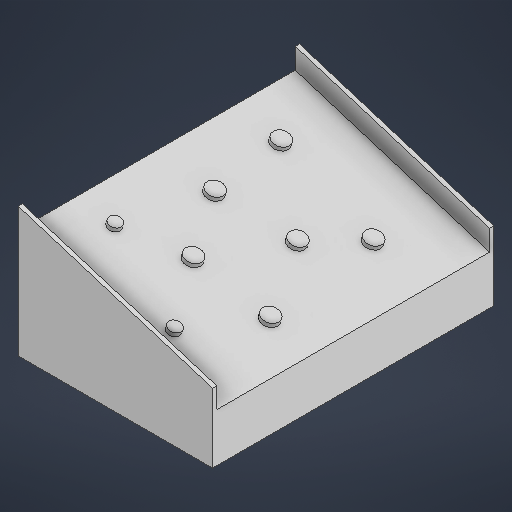
# Autodesk Inventor part: newcollection
Saved by Autodesk Inventor 2026.2 (Build 302298000, 298)
## iProperties
Created: 2026-04-15
Part Number: newcollection
Material: Generic
Document SubType Name: Modeling
Designer: danda
Density: 1 g/cm^3
Appearance: Default
Author: danda
Autodesk Inventor part; units mm, degrees
ref_plane "YZ Plane" through (0, 0, 0) normal (1, 0, 0) x (0, 1, 0)
ref_plane "XZ Plane" through (0, 0, 0) normal (0, 1, 0) x (-1, 0, 0)
ref_plane "XY Plane" through (0, 0, 0) normal (0, 0, 1) x (1, 0, 0)
sketch "Sketch1" plane through (0, 0, 0) normal (0, 0, 1) x (1, 0, 0)
  line L0 (-69.9828, 93.1946) -> (155.0172, 93.1946)
  line L1 (155.0172, 93.1946) -> (155.0172, 43.1946)
  line L2 (155.0172, 43.1946) -> (-69.9828, 43.1946)
  line L3 (-69.9828, 43.1946) -> (-69.9828, 93.1946)
  line L4 (-69.9828, 93.1946) -> (-69.9828, 163.1946)
  line L5 (-69.9828, 163.1946) -> (155.0172, 93.1946)
  line L6 (-74.9828, 93.1946) -> (-74.9828, 38.1946)
  line L7 (-74.9828, 38.1946) -> (160.0172, 38.1946)
  line L8 (160.0172, 38.1946) -> (160.0172, 96.8754)
  line L9 (-74.9828, 93.1946) -> (-74.9828, 169.9865)
  line L10 (-74.9828, 169.9865) -> (160.0172, 96.8754)
  line L11 (-69.9828, 163.1946) -> (-74.9828, 163.1946)
  line L12 (155.0172, 93.1946) -> (160.0172, 93.1946)
  line L13 (-69.9828, 93.1946) -> (-74.9828, 93.1946)
  point P0 (0, 0)
  dimension "d0" = 225
  dimension "d1" = 50
  dimension "d2" = 70
  dimension "d3" = 5
  dimension "d4" = 5
  constraints: 28 end point, 3 parallel, 3 perpendicular, 2 point on line, 1 collinear, 1 horizontal, 1 vertical, 1 other
  measures "d0" distance of L1.end L2.end
  measures "d1" distance of L0.end L1.end
  measures "d2" distance of L0.start L4.end
  measures "d3" distance between parallel lines of L3 L6
  measures "d4" distance between parallel lines of L4 L9
extrude "Extrusion1" add sketch "Sketch1" along normal blind 340 contours L13 L9 L11 L4 | L3 L2 L1 L12 L8 L7 L6 L13 | L5 L11 L9 L10 L8 L12
extrude "Extrusion2" add sketch "Sketch1" along normal blind 340 contours L4 L5 L0 | L0 L1 L2 L3
extrude "Extrusion3" cut sketch "Sketch1" along normal blind 335 contours L4 L5 L0 | L0 L1 L2 L3
extrude "Extrusion4" add sketch "Sketch1" along normal blind 5 contours L4 L5 L0 | L0 L1 L2 L3
sketch "Sketch2" plane through (-74.9828, 169.9865, 340) normal (0.2970666, 0.9548568, 0) x (0.9548568, -0.2970666, 0)
  line L0 (42.4399, 335) -> (42.4399, 5) projected
  circle A0 centre (42.4399, 75.4833) radius 7.5
  circle A1 centre (53.1004, 265.9353) radius 10
  circle A2 centre (108.208, 107.2253) radius 10
  circle A3 centre (63.1004, 176.4405) radius 10
  circle A4 centre (158.9071, 36.2466) radius 7.5
  circle A5 centre (180.5093, 255.9353) radius 10
  circle A6 centre (144.7995, 198.4836) radius 10
  circle A7 centre (195.4985, 117.2253) radius 10
  point P0 (122.0951, 340)
  dimension "d13" = 15
  dimension "d14" = 20
  dimension "d15" = 20
  dimension "d16" = 20
  dimension "d17" = 15
  dimension "d18" = 20
  dimension "d19" = 20
  dimension "d20" = 20
  constraints: 8 centre point, 1 point on line
  measures "d13" diameter of A0
  measures "d14" diameter of A1
  measures "d15" diameter of A2
  measures "d16" diameter of A3
  measures "d17" diameter of A4
  measures "d18" diameter of A5
  measures "d19" diameter of A6
  measures "d20" diameter of A7
extrude "Extrusion5" add sketch "Sketch2" along normal blind 5
sketch "Sketch3" plane through (0, 0, 340) normal (0, 0, 1) x (1, 0, 0)
  line L0 (-69.9828, 163.1946) -> (158.5319, 92.1011)
  line L1 (160.0172, 96.8754) -> (-74.9828, 169.9865) projected
  line L2 (-75.9241, 144.0974) -> (155.0172, 72.249)
  line L3 (-69.9828, 163.1946) -> (-69.9828, 142.249)
  line L4 (-69.9828, 43.1946) -> (-69.9828, 163.1946) projected
  line L5 (155.0172, 43.1946) -> (155.0172, 93.1946) projected
  line L6 (155.0172, 93.1946) -> (155.0172, 72.249)
  line L7 (-74.9828, 169.9865) -> (-74.9828, 194.9865)
  line L8 (-74.9828, 194.9865) -> (160.0172, 121.8754)
  line L9 (-69.9828, 163.1946) -> (155.0172, 93.1946) projected
  line L10 (160.0172, 96.8754) -> (160.0172, 121.8754)
  line L11 (-77.4095, 139.3231) -> (160.0172, 65.4571)
  line L12 (160.0172, 65.4571) -> (160.0172, 93.1946)
  line L13 (-69.9828, 142.249) -> (-69.9828, 137.0126)
  line L14 (155.0172, 72.249) -> (155.0172, 67.0126)
  point P0 (0, 0)
  dimension "d23" = 20
  dimension "d24" = 25
  dimension "d25" = 5
  constraints: 22 end point, 7 point on line, 4 parallel, 1 vertical, 1 other
  measures "d23" distance between parallel lines of L0 L2
  measures "d24" distance of L1.end L7.end
  measures "d25" distance between parallel lines of L2 L11
extrude "Extrusion6" add sketch "Sketch3" against normal blind 340 contours L2 L5 L11 L4
extrude "Extrusion7" add sketch "Sketch3" against normal blind 5 contours L1 L7 L8 L10
sketch "Sketch4" plane through (0, 0, 0) normal (0, 0, -1) x (-1, 0, 0)
  line L0 (74.9828, 194.9865) -> (74.9828, 38.1946) projected
  line L1 (74.9828, 169.9638) -> (74.9828, 194.9865)
  line L2 (-160.0172, 38.1946) -> (-160.0172, 121.8754) projected
  line L3 (74.9828, 194.9865) -> (-160.0172, 121.8754)
  line L4 (-160.0172, 121.8754) -> (-160.0172, 91.5878)
  line L5 (-160.0172, 96.8754) -> (74.9828, 169.9865) projected
  line L6 (74.9828, 169.9865) -> (-160.0172, 96.8754)
  point P0 (0, 0)
  constraints: 8 end point, 2 collinear, 2 point on line
extrude "Extrusion8" add sketch "Sketch4" against normal blind 5
body "Solid1"
